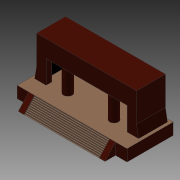
# Autodesk Inventor part: Stand
Saved by Autodesk Inventor 2015 (Build 190159000, 159)
## iProperties
Created: 2016-12-01
Part Number: Stand
Material: Generic
Document SubType Name: Modeling
Designer: Simms
Density: 1 g/cm^3
Appearance: Default
Author: Simms
Autodesk Inventor part; units mm, degrees
ref_plane "YZ Plane" through (0, 0, 0) normal (1, 0, 0) x (0, 1, 0)
ref_plane "XZ Plane" through (0, 0, 0) normal (0, 1, 0) x (-1, 0, 0)
sketch "Sketch1" plane through (0, 0, 0) normal (0, 1, 0) x (-1, 0, 0)
  line L0 (0, 0) -> (-241.3, 0)
  line L1 (-241.3, 0) -> (-241.3, -124.6632)
  line L2 (-241.3, -124.6632) -> (0, -124.6632)
  line L3 (0, -124.6632) -> (0, 0)
  dimension "d0" = 124.6632
  dimension "d1" = 241.3
  constraints: 8 end point, 2 parallel, 1 horizontal, 1 perpendicular
  measures "d0" distance of L1.end L0.end
  measures "d1" distance of L1.end L2.end
extrude "Extrusion1" add sketch "Sketch1" along normal blind 25.4
sketch "Sketch2" plane through (241.3, 0, 0) normal (1, 0, 0) x (0, 0, -1)
  line L0 (124.6632, 0) -> (226.2632, 0) construction
  line L1 (23.0632, 25.4) -> (0, 0)
  line L2 (0, 0) -> (0, 25.4)
  line L3 (0, 0) -> (0, 25.4) projected
  line L4 (0, 25.4) -> (23.0632, 25.4)
  line L5 (0, 0) -> (23.0632, 0)
  line L6 (0, 0) -> (124.6632, 0) projected
  line L7 (23.0632, 0) -> (23.0632, 25.4)
  constraints: 12 end point, 2 perpendicular, 1 collinear, 1 horizontal, 1 point on line
extrude "Extrusion2" cut sketch "Sketch2" against normal blind 25.4
ref_plane "Work Plane1" through (120.65, 0, -124.6632) normal (1, 0, 0) x (0, 0, -1)
mirror "Mirror1" about plane through (120.65, 0, -124.6632) normal (1, 0, 0) of "Extrusion2"
extrude "Extrusion3" cut sketch "Sketch2" against normal blind 228.6 contours L1 L2 L4
sketch "Sketch3" plane through (120.65, 0, -124.6632) normal (1, 0, 0) x (0, 0, -1)
  line L0 (-101.6, 25.4) -> (-101.6, 22.86)
  line L1 (-101.6, 0) -> (-101.6, 25.4) projected
  line L2 (-101.6, 22.86) -> (-104.14, 22.86)
  line L3 (-104.14, 22.86) -> (-104.14, 30.1007)
  line L4 (-104.14, 30.1007) -> (-101.6, 30.1564)
  line L5 (-101.6, 30.1564) -> (-101.6, 25.4)
  point P0 (-124.6632, 0)
  dimension "d10" = 2.54
  dimension "d11" = 2.54
  constraints: 10 end point, 1 horizontal, 1 parallel, 1 point on line, 1 vertical
  measures "d10" distance of L0.start L0.end
  measures "d11" distance of L0.end L2.end
extrude "Extrusion4" cut sketch "Sketch3" along normal mid plane 165.1
pattern_linear "Rectangular Pattern1" count 10 spacing 3.429 along (0, -0.7403, 0.6722) of "Extrusion4"
sketch "Sketch4" plane through (0, 25.4, 0) normal (0, 1, 0) x (1, 0, 0)
  line L0 (6.35, 118.3132) -> (234.95, 118.3132)
  line L1 (234.95, 118.3132) -> (234.95, 54.8132)
  line L2 (6.35, 54.8132) -> (6.35, 118.3132)
  line L3 (241.3, 23.0632) -> (241.3, 124.6632) projected
  line L4 (0, 124.6632) -> (0, 23.0632) projected
  line L5 (241.3, 124.6632) -> (0, 124.6632) projected
  line L6 (222.25, 67.5132) -> (222.25, 111.9632)
  line L7 (222.25, 111.9632) -> (19.05, 111.9632)
  line L8 (19.05, 111.9632) -> (19.05, 67.5132)
  line L9 (234.95, 54.8132) -> (222.25, 54.8132)
  line L10 (19.05, 54.8132) -> (6.35, 54.8132)
  circle A0 centre (69.85, 64.3382) radius 9.525
  circle A1 centre (171.45, 64.3382) radius 9.525
  line L11 (19.05, 54.8132) -> (31.75, 54.8132)
  line L12 (31.75, 54.8132) -> (31.75, 67.5132)
  line L13 (31.75, 67.5132) -> (19.05, 67.5132)
  line L14 (222.25, 54.8132) -> (209.55, 54.8132)
  line L15 (209.55, 54.8132) -> (209.55, 67.5132)
  line L16 (209.55, 67.5132) -> (222.25, 67.5132)
  point P0 (0, 0)
  dimension "d17" = 6.35
  dimension "d18" = 6.35
  dimension "d19" = 6.35
  dimension "d23" = 12.7
  dimension "d24" = 12.7
  dimension "d25" = 6.35
  dimension "d26" = 19.05
  dimension "d27" = 19.05
  dimension "d28" = 9.525
  dimension "d29" = 50.8
  dimension "d39" = 12.7
  dimension "d40" = 12.7
  dimension "d41" = 12.7
  dimension "d42" = 12.7
  constraints: 28 end point, 6 parallel, 3 horizontal, 3 perpendicular, 2 centre point, 1 horizontal alignment
  measures "d17" distance between parallel lines of L3 L1
  measures "d18" distance between parallel lines of L4 L2
  measures "d19" distance between parallel lines of L5 L0
  measures "d23" distance between parallel lines of L2 L8
  measures "d24" distance between parallel lines of L1 L6
  measures "d25" distance between parallel lines of L0 L7
  measures "d26" diameter of A0
  measures "d27" diameter of A1
  measures "d28" distance from line of A0.centre L10
  measures "d29" distance from line of A0.centre L8
  measures "d39" distance of L8.end L12.end
  measures "d40" distance of L12.end L11.end
  measures "d41" distance of L6.start L15.end
  measures "d42" distance of L14.end L15.end
extrude "Extrusion6" add sketch "Sketch4" along normal blind 25.4
chamfer "Chamfer1" distance 25.4 angle 10 1 edges at (234.95, 50.8, -86.5632) measured on face at (234.95, 33.8667, -97.1465)
chamfer "Chamfer2" distance 25.4 angle 10 1 edges at (6.35, 50.8, -86.5632) measured on face at (6.35, 33.8667, -75.9799)
sketch "Sketch5" plane through (0, 50.8, 0) normal (0, 1, 0) x (1, 0, 0)
  line L0 (10.8287, 54.8132) -> (10.8287, 118.3132) projected
  line L1 (10.8287, 54.8132) -> (31.75, 54.8132) projected
  line L2 (19.05, 67.5132) -> (19.05, 111.9632) projected
  line L3 (19.05, 111.9632) -> (222.25, 111.9632) projected
  line L4 (222.25, 111.9632) -> (222.25, 67.5132) projected
  line L5 (209.55, 54.8132) -> (230.4713, 54.8132) projected
  line L6 (230.4713, 118.3132) -> (230.4713, 54.8132) projected
  line L7 (230.4713, 118.3132) -> (10.8287, 118.3132) projected
  circle A0 centre (69.85, 64.3382) radius 9.525 projected
  circle A1 centre (171.45, 64.3382) radius 9.525 projected
  line L8 (31.75, 54.8132) -> (31.75, 67.5132) projected
  line L9 (31.75, 67.5132) -> (19.05, 67.5132) projected
  line L10 (222.25, 67.5132) -> (209.55, 67.5132) projected
  line L11 (209.55, 67.5132) -> (209.55, 54.8132) projected
  point P0 (0, 0)
extrude "Extrusion7" add sketch "Sketch5" along normal blind 25.4
sketch "Sketch6" plane through (0, 76.2, 0) normal (0, 1, 0) x (1, 0, 0)
  line L0 (10.8287, 118.3132) -> (230.4713, 118.3132)
  line L1 (230.4713, 118.3132) -> (230.4713, 54.8132)
  line L2 (230.4713, 54.8132) -> (10.8287, 54.8132)
  line L3 (10.8287, 54.8132) -> (10.8287, 118.3132)
  point P0 (0, 0)
  constraints: 8 end point, 2 parallel, 1 horizontal, 1 perpendicular
extrude "Extrusion8" add sketch "Sketch6" along normal blind 38.1
body "Solid1"
